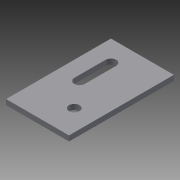
# Autodesk Inventor part: 8.2 Q1
Saved by Autodesk Inventor 2015 (Build 190159000, 159)
## iProperties
Created: 2018-04-11
Part Number: 8.2 Q1
Material: Generic
Document SubType Name: Modeling
Designer: Administrator
Density: 1 g/cm^3
Appearance: Default
Author: Administrator
Autodesk Inventor part; units mm, degrees
ref_plane "YZ Plane" through (0, 0, 0) normal (1, 0, 0) x (0, 1, 0)
ref_plane "XZ Plane" through (0, 0, 0) normal (0, 1, 0) x (-1, 0, 0)
ref_plane "XY Plane" through (0, 0, 0) normal (0, 0, 1) x (1, 0, 0)
sketch "Sketch1" plane through (0, 0, 0) normal (0, 1, 0) x (-1, 0, 0)
  line L0 (0, -127) -> (76.2, -127)
  line L1 (76.2, -127) -> (76.2, 0)
  line L2 (76.2, 0) -> (0, 0)
  line L3 (0, 0) -> (0, -127)
  line L4 (57.15, -63.5) -> (57.15, -101.6)
  line L5 (44.45, -101.6) -> (44.45, -63.5)
  arc A0 (57.15, -63.5) -> (44.45, -63.5) centre (50.8, -63.5) ccw
  arc A1 (44.45, -101.6) -> (57.15, -101.6) centre (50.8, -101.6) ccw
  circle A2 centre (25.4, -31.75) radius 6.35
  dimension "d0" = 76.2
  dimension "d2" = 127
  dimension "d3" = 38.1
  dimension "d4" = 101.6
  dimension "d5" = 25.4
  dimension "d6" = 31.75
  dimension "d7" = 50.8
  dimension "d10" = 6.35
  dimension "d11" = 6.35
  dimension "d12" = 12.7
  constraints: 12 end point, 4 point on circle, 4 tangent, 3 centre point, 3 perpendicular, 1 horizontal, 1 vertical
  measures "d0" distance of L0.start L0.end
  measures "d2" distance of L0.end L1.end
  measures "d3" distance of A1.centre A0.centre
  measures "d4" distance from line of A1.centre L2
  measures "d5" distance from line of A1.centre L1
  measures "d6" distance from line of A2.centre L2
  measures "d7" distance from line of A2.centre L1
  measures "d10" radius of A1
  measures "d11" radius of A0
  measures "d12" diameter of A2
extrude "Extrusion1" add sketch "Sketch1" along normal blind 6.35
equation "\"d2\" = 1.66667 * d0"
equation "\"d3\" = 0.5 * d0"
equation "\"d4\" = 0.8 * d2"
equation "\"d5\" = 0.333333 * d0"
equation "\"d6\" = 0.25 * d2"
equation "\"d7\" = 0.666667 * d0"
equation "\"d10\" = d8"
equation "\"d11\" = d8"
equation "\"d12\" = 2 * d8"
equation "\"d8\" = 0.05 * d2"
body "Solid1"
